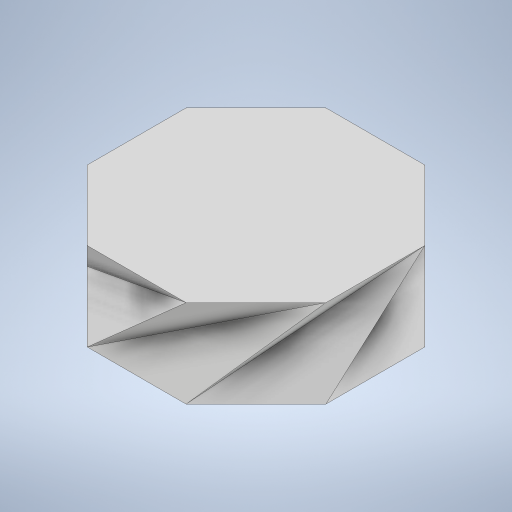
# Autodesk Inventor part: 팔각형 OV-PAM 층 한개
Saved by Autodesk Inventor 2024 (Build 280153000, 153)
## iProperties
Created: 2023-06-16
Part Number: 팔각형 OV-PAM 층 한개
Material: 일반
Document SubType Name: Modeling
Designer: jsw
Density: 1 g/cm^3
Appearance: 기본값
Author: jsw
Autodesk Inventor part; units mm, degrees
sketch "스케치1" plane through (0, 0, 0) normal (0, 1, 0) x (-1, 0, 0)
  line L0 (-31.9919, 13.2515) -> (-13.2515, 31.9919)
  line L1 (-13.2515, 31.9919) -> (13.2515, 31.9919)
  line L2 (13.2515, 31.9919) -> (31.9919, 13.2515)
  line L3 (31.9919, 13.2515) -> (31.9919, -13.2515)
  line L4 (31.9919, -13.2515) -> (13.2515, -31.9919)
  line L5 (13.2515, -31.9919) -> (-13.2515, -31.9919)
  line L6 (-13.2515, -31.9919) -> (-31.9919, -13.2515)
  line L7 (-31.9919, -13.2515) -> (-31.9919, 13.2515)
  line L8 (-13.5, 32.5919) -> (13.5, 32.5919)
  line L9 (13.5, 32.5919) -> (32.5919, 13.5)
  line L10 (32.5919, 13.5) -> (32.5919, -13.5)
  line L11 (32.5919, -13.5) -> (13.5, -32.5919)
  line L12 (13.5, -32.5919) -> (-13.5, -32.5919)
  line L13 (-13.5, -32.5919) -> (-32.5919, -13.5)
  line L14 (-32.5919, -13.5) -> (-32.5919, 13.5)
  line L15 (-32.5919, 13.5) -> (-13.5, 32.5919)
  point P0 (0, 0)
  point P1 (0, 0)
  point P2 (0, 0)
  dimension "d2" = 0.6
  dimension "d118" = 27
  constraints: 32 end point, 2 coincident, 2 horizontal, 34 other
  measures "d2" distance between parallel lines of L10 L3
  measures "d118" distance of L9.end L10.end
extrude "돌출2" add sketch "스케치1" along normal blind 24 contours L0 L1 L2 L3 L4 L5 L6 L7 | L8 L9 L10 L11 L12 L13 L14 L15
ref_plane "작업 평면24" through (-13.5, 24, -32.5919) normal (0, -0.622543, -0.7825856) x (1, 0, 0)
sketch "스케치27" plane through (13.5, 0, -32.5919) normal (0, 0, -1) x (-1, 0, 0)
  line L0 (27, 24) -> (46.0919, 24) projected
  line L1 (0, 24) -> (27, 24) projected
  line L2 (27, 24) -> (0, 24)
  line L3 (0, 24) -> (-19.0919, 0)
  line L4 (-19.0919, 0) -> (27, 24)
  line L5 (0, 0) -> (0, 24) projected
  line L6 (0, 24) -> (0, 9.9411)
  point P0 (13.5, 0)
  constraints: 8 end point, 2 point on line, 1 horizontal
extrude "돌출22" cut sketch "스케치27" against normal up to surface surface through (-13.5, 24, -32.5919) normal (0, -0.622543, -0.7825856)
ref_plane "작업 평면26" through (32.5919, 0, -13.5) normal (0.5533716, 0.622543, -0.5533716) x (-0.7071068, 0, -0.7071068)
sketch "스케치28" plane through (13.5, 0, -32.5919) normal (0.7071068, 0, -0.7071068) x (-0.7071068, 0, -0.7071068)
  line L0 (-27.3314, 0) -> (-27.3314, 12) projected
  line L1 (19.0919, 0) -> (0, 0) projected
  line L2 (-27, 0) -> (0, 0)
  line L3 (19.0919, 0) -> (19.0919, 24) projected
  line L4 (0, 0) -> (19.0919, 24)
  line L5 (19.0919, 24) -> (-27, 0)
  point P0 (-13.5, 0)
  point P1 (-27.3314, 12)
  constraints: 6 end point, 1 collinear
extrude "돌출23" cut sketch "스케치28" against normal up to surface contours L2 L5 L4 surface through (32.5919, 0, -13.5) normal (0.5533716, 0.622543, -0.5533716)
pattern_circular "원형 패턴5" count 8 over 360 about axis through (0, -10, 0) along (0, 1, 0) of "돌출23", "돌출22"
ref_plane "작업 평면27" through (0, 12, 0) normal (0, 1, 0) x (1, 0, 0)
